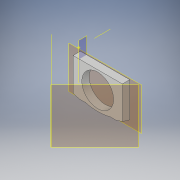
# Autodesk Inventor part: 20_Cube_Insert_Kinematic_Mirrormount_45_Thorlabsadapter
Saved by Autodesk Inventor 2019 (Build 230136000, 136)
## iProperties
Created: 2019-10-30
Part Number: 20_Cube_Insert_Kinematic_Mirrormount_45_Thorlabsadapter
Material: Generic
Document SubType Name: Modeling
Designer: diederichbenedict
Density: 1 g/cm^3
Appearance: Default
Author: diederichbenedict
Autodesk Inventor part; units mm, degrees
ref_plane "YZ Plane" through (0, 0, 0) normal (1, 0, 0) x (0, 1, 0)
ref_plane "XZ Plane" through (0, 0, 0) normal (0, 1, 0) x (-1, 0, 0)
ref_plane "Work Plane1" through (0, -12.9, 0) normal (0, 0, 1) x (1, 0, 0)
sketch "Sketch1" plane through (0, -12.9, 0) normal (0, 0, 1) x (1, 0, 0)
  circle A0 centre (26.8127, 14) radius 1.4 construction
  line L0 (6.8127, 27.5) -> (46.8127, 27.5)
  line L1 (46.8127, 27.5) -> (46.8127, 0.5)
  line L2 (46.8127, 0.5) -> (6.8127, 0.5)
  line L3 (6.8127, 0.5) -> (6.8127, 27.5)
  line L4 (6.8127, 27.5) -> (46.8127, 0.5) construction
  line L5 (46.8127, 27.5) -> (6.8127, 0.5) construction
  circle A1 centre (26.8127, 14) radius 12.7 construction
  circle A2 centre (26.8127, 14) radius 12.85
  line L6 (6.8127, 27.5) -> (46.8127, 27.5)
  line L7 (46.8127, 27.5) -> (46.8127, 28.5)
  line L8 (46.8127, 28.5) -> (6.8127, 28.5)
  line L9 (6.8127, 28.5) -> (6.8127, 27.5)
  point P0 (0, 12.9)
  dimension "d0" = 40
  dimension "d1" = 27
  dimension "d14" = 1
  dimension "d25" = 25.7
  constraints: 20 end point, 4 parallel, 2 horizontal, 2 midpoint, 2 perpendicular, 1 centre point
  measures "d0" distance of L1.end L2.end
  measures "d1" distance of L0.end L1.end
  measures "d14" distance of L7.end L6.end
  measures "d25" diameter of A2
ref_plane "Work Plane2" through (14.3627, 1.55, 6) normal (0, 0, 1) x (1, 0, 0)
extrude "Extrusion1" add sketch "Sketch1" along normal up to surface (6 mm away)
ref_plane "Work Plane3" through (11.8127, 24, 6) normal (-1, 0, 0) x (0, 0, 1)
sketch "Sketch2" plane through (11.8127, 24, 6) normal (-1, 0, 0) x (0, 0, 1)
  line L0 (-13.2187, 0) -> (3.0119, 0) projected
  line L1 (-6, -35.75) -> (-6, -10.05) projected
  line L2 (-10.9, -34.4) -> (0.6933, -34.4)
  line L3 (-10.9, -31.4) -> (0.6933, -31.4)
  line L4 (-10.9, -14.4) -> (0.6933, -14.4)
  line L5 (-10.9, -11.4) -> (0.6933, -11.4)
  arc A0 (-5.3, -10.45) -> (-5.3, -15.35) centre (-5.3, -12.9) ccw
  arc A1 (-5.4335, -30.45) -> (-5.4335, -35.35) centre (-5.4335, -32.9) ccw
  line L6 (-5.4335, -35.35) -> (-5.4335, -30.45)
  line L7 (-5.3, -15.35) -> (-5.3, -10.45)
  point P0 (-6, -24)
  dimension "d22" = 4.9
  dimension "d23" = 1.5
  dimension "d24" = 1.5
  constraints: 12 end point, 4 horizontal, 4 point on circle, 2 centre point, 1 parallel, 8 other
  measures "d22" diameter of A1
  measures "d23" distance from line of L2 A1.centre
  measures "d24" distance from line of A0.centre L4
revolve "Revolution1" cut sketch "Sketch2" angle 360 about axis through (11.8127, 8.65, 0.7) along (0, 1, 0) contours A0 L4 L1 | L1 L4 L7 A0 | L4 A0 L5 L1 | L1 L5 L7 L4 | L5 A0 L1 | L1 A0 L7 L5
pattern_linear "Rectangular Pattern1" count 2 spacing 20 along (0, -1, 0) count 2 spacing 30 along (1, 0, 0) of "Revolution1"
sketch "Sketch3" plane through (6.8127, -12.4, 6) normal (0, 0, 1) x (1, 0, 0)
  ellipse E0 centre (20, 24.3) end of major axis (41.0718, 24.3) minor radius 14.9 (7.3193, 12.4) -> (20, 9.4) ccw construction
  ellipse E1 centre (20, 24.3) end of major axis (41.0718, 24.3) minor radius 14.9 (20, 9.4) -> (32.6807, 12.4) ccw construction
  circle A0 centre (20, 13.5) radius 12.85 construction
  line L0 (40, 0) -> (0, 0) construction
  line L1 (40, 28) -> (40, 0) construction
  line L2 (0, 28) -> (40, 28) construction
  line L3 (0, 0) -> (0, 28) construction
  circle A1 centre (20, 13.5) radius 12.85 construction
  line L4 (40, 0) -> (0, 0) projected
  line L5 (10.0003, 0) -> (29.9997, 0)
  spline S0 degree 5 poles (2.3021, 2.9833) (5.5467, 1.2547) (9.0339, -0.0186) (12.6471, -0.8521) (16.3235, -1.2698) (20, -1.2699) knots 0 0 0 0 0 0 1 1 1 1 1 1
  spline S1 degree 5 poles (20, -1.2699) (23.6765, -1.2698) (27.3529, -0.8521) (30.9661, -0.0186) (34.4533, 1.2547) (37.6979, 2.9833) knots 0 0 0 0 0 0 1 1 1 1 1 1
  point P0 (-6.8127, 12.4)
  constraints: 2 end point, 2 point on line, 10 other
extrude "Extrusion2" add sketch "Sketch3" against normal up to surface (6 mm away)
ref_plane "Work Plane4" through (26.8127, 23.9, 43.6151) normal (-0.7071068, 0, 0.7071068) x (-0.7071068, 0, -0.7071068)
sketch "Sketch4" plane through (26.8127, 23.9, 43.6151) normal (-0.7071068, 0, 0.7071068) x (-0.7071068, 0, -0.7071068)
  arc A0 (33.8666, 23.9) -> (15.9334, 23.9) centre (24.9, 12) ccw projected
  ellipse E0 centre (26.5979, 22.8) end of major axis (26.5979, 35.65) minor radius 9.0863 construction
  line L0 (12.4558, 36.3) -> (19.5271, 36.3) construction
  line L1 (12.4558, 8.3) -> (12.4558, 36.3) construction
  line L2 (40.74, 8.3) -> (12.4558, 8.3) construction
  line L3 (40.74, 36.3) -> (40.74, 8.3) construction
  line L4 (33.6687, 36.3) -> (40.74, 36.3) projected
  arc A1 (33.5545, 36.3) -> (9.1298, 32.4131) centre (24.9, 12) ccw
  line L5 (33.6687, 36.3) -> (40.74, 36.3) projected
  line L6 (33.5545, 36.3) -> (40.74, 36.3)
  line L7 (40.74, 36.3) -> (40.74, 42.5179)
  line L8 (40.74, 42.5179) -> (9.2813, 42.9694)
  line L9 (9.2813, 42.9694) -> (9.1298, 32.4131)
  point P0 (49.8, 23.9)
  constraints: 8 end point, 2 perpendicular, 2 point on circle, 1 centre point, 1 horizontal, 3 other
extrude "Extrusion3" cut sketch "Sketch4" against normal through all
ref_plane "Work Plane5" through (62.0266, 23.9, 8.4012) normal (0.7071068, 0, 0.7071068) x (-0.7071068, 0, 0.7071068)
sketch "Sketch5" plane through (62.0266, 23.9, 8.4012) normal (0.7071068, 0, 0.7071068) x (-0.7071068, 0, 0.7071068)
  arc A0 (33.8666, 23.9) -> (15.9334, 23.9) centre (24.9, 12) ccw projected
  arc A1 (40.4723, 32.6668) -> (9.3277, 32.6668) centre (24.9, 12) ccw
  line L0 (16.1313, 36.3) -> (11.8886, 36.3) projected
  line L1 (16.1313, 36.3) -> (16.2449, 36.3865) construction
  line L2 (16.2449, 36.3865) -> (16.1313, 36.3)
  line L3 (40.4723, 32.6668) -> (40.4723, 41.9024)
  line L4 (40.4723, 41.9024) -> (12.0732, 41.9024)
  line L5 (12.0732, 41.9024) -> (11.8886, 36.3)
  point P0 (37.9189, 23.9)
  constraints: 10 end point, 3 point on circle, 1 centre point, 1 collinear, 1 perpendicular, 1 vertical
extrude "Extrusion4" cut sketch "Sketch5" against normal through all
body "Solid1"
